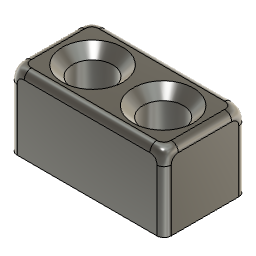
photo_support (Autodesk Fusion 360 design; units mm, degrees)
Autodesk Fusion 360 part; units mm, degrees
sketch "Sketch1" plane through (0, 0, 0) normal (0, 0, 1) x (1, 0, 0)
  line L0 (-10.3572, 16.2336) -> (20.1833, 16.2336)
  line L1 (20.1833, 16.2336) -> (20.1833, 0)
  line L2 (20.1833, 0) -> (-10.3572, 0)
  line L3 (-10.3572, 0) -> (-10.3572, 16.2336)
  circle A0 centre (-2, 8) radius 1.5
  circle A1 centre (12, 8) radius 1.5
  dimension "d1" = 3
  dimension "d2" = 3
  constraint horizontal L0
  constraint vertical L1
  constraint horizontal L2
  constraint vertical L3
  measures "d1" diameter of A0
  measures "d2" diameter of A1
extrude "Extrude1" add sketch "Sketch1" along normal blind 15
hole "Hole3" at (12, 8, 15) direction (0, 0, -1) diameter 8 depth 10 tip angle 118 countersink diameter 12 countersink angle 90
hole "Hole4" at (-2, 8, 15) direction (0, 0, -1) diameter 8 depth 10 tip angle 118 countersink diameter 12 countersink angle 90
fillet "Fillet2" chord length 2 8 edges at (4.913, 0, 15) (-10.3572, 8.1168, 15) (4.913, 16.2336, 15) (20.1833, 8.1168, 15) (20.1833, 0, 7.5) (-10.3572, 0, 7.5) (-10.3572, 16.2336, 7.5) (20.1833, 16.2336, 7.5)
